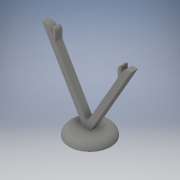
# Autodesk Inventor part: mask holder
Saved by Autodesk Inventor 2019.2 (Build 232265000, 265)
## iProperties
Created: 2020-09-18
Part Number: mask holder
Material: Rubber
Document SubType Name: Modeling
Designer: SnoBotics
Density: 0.93 g/cm^3
Appearance: Rubber - Black
Author: SnoBotics
Autodesk Inventor part; units mm, degrees
ref_plane "YZ Plane" through (0, 0, 0) normal (1, 0, 0) x (0, 1, 0)
ref_plane "XZ Plane" through (0, 0, 0) normal (0, 1, 0) x (-1, 0, 0)
ref_plane "XY Plane" through (0, 0, 0) normal (0, 0, 1) x (1, 0, 0)
sketch "Sketch1" plane through (0, 0, 0) normal (0, 0, 1) x (1, 0, 0)
  line L0 (0, 0) -> (6.35, 0)
  line L1 (0, 0) -> (-6.3448, 0)
  line L2 (6.35, 0) -> (82.5616, 131.9842)
  line L3 (82.5616, 131.9842) -> (69.8518, 131.9842)
  line L4 (69.8518, 131.9842) -> (0.0026, 10.9947)
  line L5 (0.0026, 10.9947) -> (-69.8461, 131.9845)
  line L6 (-6.3448, 0) -> (-82.5554, 131.9845)
  line L7 (-82.5554, 131.9845) -> (-69.8461, 131.9845)
  dimension "d2" = 6.35
  constraints: 16 end point, 3 horizontal
  measures "d2" distance of L0.start L0.end
extrude "Extrusion1" add sketch "Sketch1" along normal blind 12.7
sketch "Sketch2" plane through (-6.3448, 0, 0) normal (0, -1, 0) x (1, 0, 0)
  circle A0 centre (6.3474, 6.35) radius 38.1
  point P0 (6.3448, 0)
  dimension "d7" = 76.2
  constraints: 1 centre point
  measures "d7" diameter of A0
extrude "Extrusion2" add sketch "Sketch2" along normal blind 12.7
fillet "Fillet1" radius 12.7 1 edges at (-38.0974, 0, 6.35)
fillet "Fillet2" radius 2.8575 1 edges at (0.0026, 10.9947, 6.35)
sketch "Sketch4" plane through (0, 0, 12.7) normal (0, 0, 1) x (1, 0, 0)
  line L0 (82.5616, 131.9842) -> (69.8518, 131.9842) construction
  line L1 (69.8518, 131.9842) -> (2.4773, 15.2813) construction
  line L2 (63.5021, 120.9855) -> (63.5021, 131.9842)
  line L3 (63.5021, 131.9842) -> (57.7871, 131.9842)
  line L4 (57.7871, 131.9842) -> (57.7871, 111.0863)
  line L5 (-63.5021, 120.9855) -> (-63.5021, 131.9842)
  line L6 (-63.5021, 131.9842) -> (-57.7871, 131.9842)
  line L7 (-57.7871, 131.9842) -> (-57.7871, 111.0862)
  line L8 (-63.5021, 120.9855) -> (-57.7871, 111.0862)
  line L9 (-2.4721, 15.2813) -> (-69.8461, 131.9845) projected
  line L10 (57.7871, 111.0863) -> (63.5021, 120.9855)
  point P0 (0, 0)
  dimension "d19" = 12.7
  dimension "d20" = 5.715
  constraints: 16 end point, 2 point on line, 1 collinear, 1 horizontal, 1 parallel, 1 perpendicular, 1 vertical
  measures "d19" distance of L0.end L2.start
  measures "d20" distance of L2.end L3.end
extrude "Extrusion4" add sketch "Sketch4" against normal blind 12.7
fillet "Fillet5" radius 5.3975 2 edges at (57.7871, 131.9842, 6.35) (-57.7871, 131.9842, 6.35)
fillet "Fillet6" radius 13.335 2 edges at (69.8518, 131.9842, 6.35) (-69.8461, 131.9845, 6.35)
body "Solid1"
